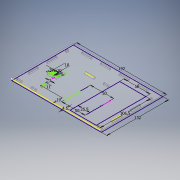
# Autodesk Inventor part: base_v2
Saved by Autodesk Inventor 2017.2 (Build 212233000, 233)
## iProperties
Created: 2017-06-08
Part Number: base_v2
Material: Generic
Document SubType Name: Modeling
Designer: SandeepSH
Density: 1 g/cm^3
Appearance: Polycarbonate - Clear
Author: SandeepSH
Autodesk Inventor part; units mm, degrees
ref_plane "YZ Plane" through (0, 0, 0) normal (1, 0, 0) x (0, 1, 0)
ref_plane "XZ Plane" through (0, 0, 0) normal (0, 1, 0) x (-1, 0, 0)
ref_plane "XY Plane" through (0, 0, 0) normal (0, 0, 1) x (1, 0, 0)
sketch "Sketch1" plane through (0, 0, 0) normal (0, 1, 0) x (-1, 0, 0)
  line L0 (0, 0) -> (-192, 0)
  line L1 (-192, 0) -> (-192, -132)
  line L2 (-192, -132) -> (0, -132)
  line L3 (0, -132) -> (0, 0)
  dimension "d0" = 192
  dimension "d1" = 132
  constraints: 8 end point, 2 parallel, 1 horizontal, 1 perpendicular
  measures "d0" distance of L2.end L1.end
  measures "d1" distance of L1.end L0.end
extrude "Extrusion1" add sketch "Sketch1" along normal blind 3
fillet "Fillet1" radius 2 4 edges at (0, 1.5, 0) (192, 1.5, 0) (0, 1.5, -132) (192, 1.5, -132) curvature continuous yes
sketch "Sketch2" plane through (0, 3, 0) normal (0, 1, 0) x (1, 0, 0)
  point P0 (0, 0)
sketch "Sketch3" plane through (0, 3, 0) normal (0, 1, 0) x (1, 0, 0)
  line L0 (26, 127) -> (46, 127)
  line L1 (46, 127) -> (46, 124)
  line L2 (46, 124) -> (26, 124)
  line L3 (26, 124) -> (26, 127)
  line L4 (190, 132) -> (2, 132) projected
  line L5 (0, 130) -> (0, 2) projected
  line L6 (66, 127) -> (86, 127)
  line L7 (86, 127) -> (86, 124)
  line L8 (86, 124) -> (66, 124)
  line L9 (66, 124) -> (66, 127)
  line L10 (106, 127) -> (126, 127)
  line L11 (126, 127) -> (126, 124)
  line L12 (126, 124) -> (106, 124)
  line L13 (106, 124) -> (106, 127)
  line L14 (146, 124) -> (166, 124)
  line L15 (166, 124) -> (166, 127)
  line L16 (166, 127) -> (146, 127)
  line L17 (146, 127) -> (146, 124)
  point P0 (0, 0)
  dimension "d5" = 20
  dimension "d6" = 3
  dimension "d7" = 5
  dimension "d8" = 26
  dimension "d9" = 20
  dimension "d10" = 3
  dimension "d11" = 20
  dimension "d12" = 20
  dimension "d13" = 20
  dimension "d14" = 3
  dimension "d15" = 20
  dimension "d16" = 20
  dimension "d20" = 3
  constraints: 32 end point, 8 parallel, 4 horizontal, 4 perpendicular, 3 collinear
  measures "d5" distance of L1.end L2.end
  measures "d6" distance of L0.end L1.end
  measures "d7" distance between parallel lines of L4 L0
  measures "d8" distance between parallel lines of L3 L5
  measures "d9" distance of L7.end L8.end
  measures "d10" distance between parallel lines of L6 L8
  measures "d11" distance between parallel lines of L1 L9
  measures "d12" distance of L11.end L12.end
  measures "d13" distance between parallel lines of L7 L13
  measures "d14" distance between parallel lines of L10 L12
  measures "d15" distance of L16.end L15.end
  measures "d16" distance between parallel lines of L17 L11
  measures "d20" distance between parallel lines of L14 L16
sketch "Sketch4" plane through (0, 3, 0) normal (0, 1, 0) x (1, 0, 0)
  line L0 (5, 30) -> (8, 30)
  line L1 (8, 30) -> (8, 50)
  line L2 (8, 50) -> (5, 50)
  line L3 (5, 50) -> (5, 30)
  line L4 (2, 0) -> (190, 0) projected
  line L5 (5, 70) -> (8, 70)
  line L6 (8, 70) -> (8, 90)
  line L7 (8, 90) -> (5, 90)
  line L8 (5, 90) -> (5, 70)
  line L9 (5, 110) -> (8, 110)
  line L10 (8, 110) -> (8, 115)
  line L11 (8, 115) -> (5, 115)
  line L12 (5, 115) -> (5, 110)
  line L13 (0, 130) -> (0, 2) projected
  line L14 (96, 70) -> (96, 132)
  line L15 (190, 132) -> (2, 132) projected
  line L16 (187, 30) -> (184, 30)
  line L17 (184, 30) -> (184, 50)
  line L18 (184, 50) -> (187, 50)
  line L19 (187, 50) -> (187, 30)
  line L20 (187, 70) -> (184, 70)
  line L21 (184, 70) -> (184, 90)
  line L22 (184, 90) -> (187, 90)
  line L23 (187, 90) -> (187, 70)
  line L24 (187, 110) -> (184, 110)
  line L25 (184, 110) -> (184, 115)
  line L26 (184, 115) -> (187, 115)
  line L27 (187, 115) -> (187, 110)
  line L28 (192, 2) -> (192, 130) projected
  point P0 (0, 0)
  dimension "d23" = 3
  dimension "d24" = 20
  dimension "d25" = 30
  dimension "d26" = 3
  dimension "d27" = 20
  dimension "d28" = 20
  dimension "d29" = 5
  dimension "d30" = 20
  dimension "d31" = 96
  dimension "d72" = 5
  dimension "d73" = 3
  dimension "d85" = 192
  constraints: 50 end point, 12 symmetric about line, 6 parallel, 3 horizontal, 3 perpendicular, 2 collinear, 1 midpoint
  measures "d23" distance of L2.end L1.end
  measures "d24" distance of L1.end L0.end
  measures "d25" distance between parallel lines of L4 L0
  measures "d26" distance of L7.end L6.end
  measures "d27" distance of L6.end L5.end
  measures "d28" distance between parallel lines of L5 L2
  measures "d29" distance of L10.end L9.end
  measures "d30" distance between parallel lines of L9 L7
  measures "d31" distance from line of L13 L14.start
  measures "d72" distance between parallel lines of L13 L8
  measures "d73" distance between parallel lines of L12 L10
  measures "d85" distance between parallel lines of L28 L13
extrude "Extrusion3" cut sketch "Sketch4" against normal through all
sketch "Sketch5" plane through (0, 3, 0) normal (0, 1, 0) x (1, 0, 0)
  line L0 (184, 30) -> (184, 50) projected
  line L1 (2, 0) -> (190, 0) projected
  line L2 (96, 70) -> (96, 17.3538)
  line L3 (46, 50) -> (43, 50)
  line L4 (43, 50) -> (43, 70)
  line L5 (43, 70) -> (46, 70)
  line L6 (46, 70) -> (46, 50)
  line L7 (43, 19) -> (46, 19)
  line L8 (46, 19) -> (46, 30)
  line L9 (46, 30) -> (43, 30)
  line L10 (43, 30) -> (43, 19)
  point P0 (0, 0)
  dimension "d57" = 3
  dimension "d58" = 11
  dimension "d59" = 19
  constraints: 18 end point, 2 collinear, 2 parallel, 1 horizontal, 1 perpendicular, 1 vertical
  measures "d57" distance of L9.end L8.end
  measures "d58" distance of L8.end L7.end
  measures "d59" distance between parallel lines of L1 L7
sketch "Sketch6" plane through (0, 3, 0) normal (0, 1, 0) x (1, 0, 0)
  line L0 (187, 5) -> (179, 5)
  line L1 (179, 5) -> (179, 8)
  line L2 (179, 8) -> (187, 8)
  line L3 (187, 8) -> (187, 5)
  line L4 (2, 0) -> (190, 0) projected
  line L5 (192, 2) -> (192, 130) projected
  line L6 (5, 5) -> (15, 5)
  line L7 (15, 5) -> (15, 8)
  line L8 (15, 8) -> (5, 8)
  line L9 (5, 8) -> (5, 5)
  line L10 (0, 130) -> (0, 2) projected
  line L11 (36, 5) -> (46, 5)
  line L12 (46, 5) -> (46, 8)
  line L13 (46, 8) -> (36, 8)
  line L14 (36, 8) -> (36, 5)
  line L15 (46, 30) -> (46, 19) projected
  point P0 (0, 0)
  dimension "d46" = 8
  dimension "d47" = 3
  dimension "d48" = 5
  dimension "d49" = 5
  dimension "d50" = 10
  dimension "d51" = 3
  dimension "d52" = 5
  dimension "d53" = 5
  dimension "d60" = 10
  dimension "d61" = 3
  constraints: 24 end point, 6 parallel, 3 horizontal, 3 perpendicular, 2 collinear
  measures "d46" distance of L1.end L2.end
  measures "d47" distance of L0.end L1.end
  measures "d48" distance between parallel lines of L4 L0
  measures "d49" distance between parallel lines of L5 L3
  measures "d50" distance of L8.end L7.end
  measures "d51" distance of L7.end L6.end
  measures "d52" distance between parallel lines of L10 L9
  measures "d53" distance between parallel lines of L4 L6
  measures "d60" distance of L13.end L12.end
  measures "d61" distance of L12.end L11.end
sketch "Sketch7" plane through (0, 3, 0) normal (0, 1, 0) x (1, 0, 0)
  line L0 (66, 90) -> (86, 90)
  line L1 (86, 90) -> (86, 93)
  line L2 (86, 93) -> (66, 93)
  line L3 (66, 93) -> (66, 90)
  line L4 (43, 90) -> (46, 90) projected
  line L5 (46, 90) -> (46, 80) projected
  line L6 (106, 90) -> (116, 90)
  line L7 (116, 90) -> (116, 93)
  line L8 (116, 93) -> (106, 93)
  line L9 (106, 93) -> (106, 90)
  line L10 (146, 80) -> (146, 90) projected
  point P0 (0, 0)
  dimension "d64" = 20
  dimension "d65" = 3
  dimension "d66" = 20
  dimension "d67" = 10
  dimension "d68" = 3
  dimension "d69" = 30
  constraints: 16 end point, 4 parallel, 2 collinear, 2 horizontal, 2 perpendicular
  measures "d64" distance of L2.end L1.end
  measures "d65" distance of L1.end L0.end
  measures "d66" distance between parallel lines of L3 L5
  measures "d67" distance of L8.end L7.end
  measures "d68" distance of L7.end L6.end
  measures "d69" distance between parallel lines of L7 L10
extrude "Extrusion6" cut sketch "Sketch7" against normal through all
sketch "Sketch8" plane through (0, 3, 0) normal (0, 1, 0) x (1, 0, 0)
  line L0 (86, 90) -> (66, 90) projected
  line L1 (43, 65) -> (43, 45) projected
  line L2 (38, 56.5) -> (38, 53.5)
  line L3 (38, 53.5) -> (28, 53.5)
  line L4 (28, 53.5) -> (28, 56.5)
  line L5 (28, 56.5) -> (38, 56.5)
  line L6 (38, 56.5) -> (28, 53.5) construction
  line L7 (38, 53.5) -> (28, 56.5) construction
  line L8 (96, 67.642) -> (96, 32.7104)
  line L9 (146, 45) -> (146, 65) projected
  line L10 (28, 58.5) -> (38, 58.5)
  line L11 (38, 58.5) -> (38, 61.5)
  line L12 (38, 61.5) -> (28, 61.5)
  line L13 (28, 61.5) -> (28, 58.5)
  line L14 (28, 51.5) -> (38, 51.5)
  line L15 (38, 51.5) -> (38, 48.5)
  line L16 (38, 48.5) -> (28, 48.5)
  line L17 (28, 48.5) -> (28, 51.5)
  point P0 (0, 0)
  point P1 (43, 55)
  point P2 (33, 55)
  dimension "d75" = 5
  dimension "d76" = 10
  dimension "d77" = 50
  dimension "d78" = 3
  dimension "d80" = 10
  dimension "d81" = 3
  dimension "d82" = 2
  constraints: 30 end point, 4 parallel, 3 midpoint, 2 perpendicular, 2 vertical, 1 collinear, 1 horizontal
  measures "d75" distance between parallel lines of L1 L2
  measures "d76" distance between parallel lines of L2 L4
  measures "d77" distance between parallel lines of L9 L8
  measures "d78" distance between parallel lines of L3 L5
  measures "d80" distance of L12.end L11.end
  measures "d81" distance of L11.end L10.end
  measures "d82" distance between parallel lines of L10 L5
extrude "Extrusion7" [suppressed]
sketch "arduino" plane through (0, 3, 0) normal (0, 1, 0) x (1, 0, 0)
  line L0 (55, 137) -> (35, 137) projected
  line L1 (35, 137) -> (5.0623, 137)
  line L2 (8, 115) -> (8, 110) projected
  line L3 (8, 118.6544) -> (8, 143.1014)
  line L4 (8, 137) -> (62, 137)
  line L5 (62, 137) -> (62, 66)
  line L6 (62, 66) -> (8, 66)
  line L7 (8, 66) -> (8, 137)
  line L8 (30.5, 71.242) -> (30.5, 18.397)
  line L9 (46, 65) -> (46, 45) projected
  line L10 (25.5, 71.242) -> (25.5, 36.8941)
  line L11 (46, 124) -> (26, 124) projected
  line L12 (13, 124) -> (84, 124)
  line L13 (84, 124) -> (84, 70)
  line L14 (84, 70) -> (13, 70)
  line L15 (13, 70) -> (13, 124)
  line L16 (13, 115) -> (16, 115)
  line L17 (16, 115) -> (16, 103)
  line L18 (16, 103) -> (13, 103)
  line L19 (13, 103) -> (13, 115)
  point P0 (0, 0)
  dimension "d86" = 54
  dimension "d87" = 71
  dimension "d88" = 15.5
  dimension "d89" = 5
  dimension "d92" = 71
  dimension "d93" = 54
  dimension "d94" = 3
  dimension "d95" = 12
  dimension "d96" = 9
  constraints: 32 end point, 6 parallel, 4 horizontal, 4 perpendicular, 4 point on line, 2 vertical, 1 collinear
  measures "d86" distance of L5.end L6.end
  measures "d87" distance of L4.end L5.end
  measures "d88" distance between parallel lines of L9 L8
  measures "d89" distance between parallel lines of L8 L10
  measures "d92" distance of L13.end L14.end
  measures "d93" distance of L12.end L13.end
  measures "d94" distance of L17.end L18.end
  measures "d95" distance of L16.end L17.end
  measures "d96" distance between parallel lines of L12 L16
extrude "Extrusion8" cut sketch "Sketch6" against normal through all
extrude "Extrusion9" cut sketch "Sketch3" against normal through all
extrude "Extrusion10" [suppressed]
extrude "Extrusion11" cut sketch "Sketch5" against normal through all
extrude "Extrusion12" cut sketch "Sketch8" against normal through all
sketch "Sketch10" plane through (0, 3, 0) normal (0, 1, 0) x (1, 0, 0)
  line L0 (120.5, 4.5) -> (176.5, 4.5)
  line L1 (176.5, 4.5) -> (176.5, 111)
  line L2 (176.5, 111) -> (120.5, 111)
  line L3 (120.5, 111) -> (120.5, 4.5)
  line L4 (146, 50.0185) -> (146, 14.3687)
  line L5 (96, 70) -> (96, 17.3538) projected
  line L6 (2, 0) -> (190, 0) projected
  point P0 (0, 0)
  dimension "d105" = 56
  dimension "d106" = 106.5
  dimension "d107" = 50
  dimension "d108" = 25.5
  dimension "d109" = 4.5
  constraints: 10 end point, 2 parallel, 1 horizontal, 1 perpendicular, 1 vertical
  measures "d105" distance of L2.end L1.end
  measures "d106" distance of L1.end L0.end
  measures "d107" distance between parallel lines of L4 L5
  measures "d108" distance between parallel lines of L4 L3
  measures "d109" distance between parallel lines of L6 L0
equation "\"d9\" = d5"
equation "\"d10\" = d6"
equation "\"d11\" = d5"
equation "\"d12\" = d5"
equation "\"d13\" = d9"
equation "\"d14\" = d10"
equation "\"d15\" = d16"
equation "\"d16\" = d12"
equation "\"d20\" = d14"
equation "\"d31\" = 0.5 * d85"
equation "\"d53\" = d48"
equation "\"d66\" = d64"
equation "\"d80\" = d76"
body "Solid1"
